Autodesk Inventor part; units mm, degrees
(part 9 of 16)
  spline S53 degree 3 poles (39.1598, 73.1537) (39.0289, 73.1211) (38.8976, 73.0905) (38.7657, 73.0621) (38.6945, 73.0467) (38.6231, 73.0319) (38.5516, 73.0177) (38.4838, 73.0044) (38.416, 72.9916) (38.3481, 72.9794) (38.284, 72.9679) (38.2197, 72.957) (38.1554, 72.9466) (38.095, 72.9369) (38.0344, 72.9277) (37.9738, 72.919) (37.917, 72.9109) (37.8601, 72.9033) (37.8032, 72.8962) (37.7501, 72.8896) (37.697, 72.8834) (37.6438, 72.8778) (37.5945, 72.8725) (37.5452, 72.8677) (37.4958, 72.8633) (37.4502, 72.8593) (37.4047, 72.8556) (37.3591, 72.8524) (37.3174, 72.8494) (37.2756, 72.8469) (37.2339, 72.8446) (37.196, 72.8426) (37.1581, 72.841) (37.1202, 72.8396) (37.0861, 72.8384) (37.0521, 72.8375) (37.0181, 72.8369) (36.9731, 72.8362) (36.9281, 72.8361) (36.8831, 72.8364) (36.873, 72.8364) (36.863, 72.8365) (36.8529, 72.8365) (36.8431, 72.8364) (36.8332, 72.8363) (36.8234, 72.8361) (36.8138, 72.8359) (36.8041, 72.8356) (36.7945, 72.8352) (36.7851, 72.8348) (36.7757, 72.8344) (36.7662, 72.8338) (36.757, 72.8333) (36.7477, 72.8327) (36.7385, 72.8319) (36.7294, 72.8312) (36.7203, 72.8304) (36.7113, 72.8295) (36.7023, 72.8286) (36.6933, 72.8276) (36.6844, 72.8265) (36.6756, 72.8254) (36.6667, 72.8242) (36.6579, 72.8229) (36.6491, 72.8216) (36.6403, 72.8201) (36.6316, 72.8186) (36.6228, 72.817) (36.6141, 72.8153) (36.6054, 72.8135) (36.5966, 72.8116) (36.5878, 72.8097) (36.5791, 72.8075) (36.5702, 72.8053) (36.5613, 72.803) (36.5525, 72.8005) (36.5435, 72.7979) (36.5345, 72.7952) (36.5255, 72.7922) (36.5162, 72.7892) (36.507, 72.7859) (36.4978, 72.7824) (36.4882, 72.7787) (36.4786, 72.7748) (36.4692, 72.7706) (36.459, 72.7661) (36.449, 72.7613) (36.4392, 72.7562) (36.4285, 72.7507) (36.418, 72.7448) (36.4078, 72.7385) (36.3964, 72.7316) (36.3854, 72.7242) (36.3747, 72.7164) (36.3627, 72.7077) (36.3511, 72.6984) (36.3401, 72.6885) (36.3276, 72.6775) (36.3157, 72.6658) (36.3046, 72.6534) (36.2921, 72.6395) (36.2804, 72.6248) (36.2698, 72.6094) (36.258, 72.5923) (36.2474, 72.5743) (36.2382, 72.5556) (36.2281, 72.5354) (36.2197, 72.5143) (36.2132, 72.4928) (36.207, 72.4721) (36.2027, 72.451) (36.1987, 72.4298) (36.1788, 72.3251) (36.168, 72.219) (36.1519, 72.1138) (36.1359, 72.0085) (36.1147, 71.904) (36.1024, 71.7981) (36.0999, 71.7767) (36.0978, 71.7552) (36.0976, 71.7337) (36.0973, 71.7112) (36.0991, 71.6886) (36.1026, 71.6663) (36.1059, 71.6457) (36.1106, 71.6254) (36.1168, 71.6055) (36.1224, 71.5877) (36.1291, 71.5702) (36.1369, 71.5532) (36.1439, 71.538) (36.1517, 71.5233) (36.1603, 71.509) (36.168, 71.4963) (36.1763, 71.484) (36.1851, 71.4721) (36.193, 71.4615) (36.2013, 71.4511) (36.2101, 71.4412) (36.218, 71.4321) (36.2263, 71.4234) (36.2348, 71.4149) (36.2427, 71.4071) (36.2508, 71.3995) (36.2591, 71.3922) (36.2669, 71.3854) (36.2749, 71.3788) (36.283, 71.3724) (36.2907, 71.3664) (36.2985, 71.3605) (36.3065, 71.3548) (36.3142, 71.3493) (36.3219, 71.344) (36.3298, 71.3389) (36.3375, 71.3338) (36.3452, 71.329) (36.3531, 71.3243) (36.3608, 71.3196) (36.3685, 71.3151) (36.3764, 71.3107) (36.3842, 71.3064) (36.392, 71.3022) (36.3999, 71.2981) (36.4078, 71.294) (36.4157, 71.29) (36.4237, 71.2861) (36.4318, 71.2822) (36.4398, 71.2785) (36.448, 71.2748) (36.4562, 71.2711) (36.4644, 71.2674) (36.4727, 71.2639) (36.4811, 71.2603) (36.4895, 71.2569) (36.498, 71.2535) (36.5066, 71.25) (36.5152, 71.2467) (36.5239, 71.2434) (36.5327, 71.2401) (36.5416, 71.2368) (36.5505, 71.2337) (36.5595, 71.2304) (36.5686, 71.2273) (36.5778, 71.2242) (36.5871, 71.2211) (36.5965, 71.218) (36.6058, 71.2151) (36.6154, 71.2121) (36.6251, 71.2091) (36.6347, 71.2062) (36.6777, 71.193) (36.7207, 71.1795) (36.7634, 71.1654) (36.7957, 71.1548) (36.8279, 71.1437) (36.86, 71.1325) (36.8958, 71.1199) (36.9315, 71.107) (36.9671, 71.0938) (37.0063, 71.0793) (37.0454, 71.0643) (37.0843, 71.0491) (37.1269, 71.0324) (37.1693, 71.0154) (37.2115, 70.998) (37.2574, 70.9791) (37.3031, 70.9598) (37.3486, 70.9401) (37.3976, 70.9188) (37.4465, 70.8971) (37.4952, 70.875) (37.5474, 70.8513) (37.5995, 70.8271) (37.6512, 70.8024) (37.7066, 70.7761) (37.7616, 70.7493) (37.8165, 70.722) (37.8748, 70.693) (37.9328, 70.6634) (37.9906, 70.6333) (38.0518, 70.6015) (38.1128, 70.5691) (38.1734, 70.5361) (38.2375, 70.5013) (38.3012, 70.4659) (38.3647, 70.43) (38.482, 70.3636) (38.5983, 70.2952) (38.7136, 70.2252) knots 0 0 0 0 0.057795 0.057795 0.057795 0.089038 0.089038 0.089038 0.118617 0.118617 0.118617 0.14653 0.14653 0.14653 0.172778 0.172778 0.172778 0.19736 0.19736 0.19736 0.220277 0.220277 0.220277 0.241529 0.241529 0.241529 0.261115 0.261115 0.261115 0.279036 0.279036 0.279036 0.295292 0.295292 0.295292 0.309882 0.309882 0.309882 0.329164 0.329164 0.329164 0.333477 0.333477 0.333477 0.337694 0.337694 0.337694 0.34182 0.34182 0.34182 0.345864 0.345864 0.345864 0.349834 0.349834 0.349834 0.353742 0.353742 0.353742 0.3576 0.3576 0.3576 0.361424 0.361424 0.361424 0.365232 0.365232 0.365232 0.369048 0.369048 0.369048 0.372899 0.372899 0.372899 0.376819 0.376819 0.376819 0.380853 0.380853 0.380853 0.385052 0.385052 0.385052 0.389482 0.389482 0.389482 0.394225 0.394225 0.394225 0.399381 0.399381 0.399381 0.405067 0.405067 0.405067 0.411413 0.411413 0.411413 0.418548 0.418548 0.418548 0.426565 0.426565 0.426565 0.435472 0.435472 0.435472 0.445133 0.445133 0.445133 0.45436 0.45436 0.45436 0.5 0.5 0.5 0.54564 0.54564 0.54564 0.554867 0.554867 0.554867 0.564528 0.564528 0.564528 0.573435 0.573435 0.573435 0.581452 0.581452 0.581452 0.588587 0.588587 0.588587 0.594933 0.594933 0.594933 0.600619 0.600619 0.600619 0.605775 0.605775 0.605775 0.610518 0.610518 0.610518 0.614948 0.614948 0.614948 0.619147 0.619147 0.619147 0.623181 0.623181 0.623181 0.627101 0.627101 0.627101 0.630952 0.630952 0.630952 0.634768 0.634768 0.634768 0.638576 0.638576 0.638576 0.6424 0.6424 0.6424 0.646258 0.646258 0.646258 0.650166 0.650166 0.650166 0.654136 0.654136 0.654136 0.65818 0.65818 0.65818 0.662306 0.662306 0.662306 0.666523 0.666523 0.666523 0.670836 0.670836 0.670836 0.690118 0.690118 0.690118 0.704708 0.704708 0.704708 0.720964 0.720964 0.720964 0.738885 0.738885 0.738885 0.758471 0.758471 0.758471 0.779723 0.779723 0.779723 0.80264 0.80264 0.80264 0.827222 0.827222 0.827222 0.85347 0.85347 0.85347 0.881383 0.881383 0.881383 0.910962 0.910962 0.910962 0.942205 0.942205 0.942205 1 1 1 1
  arc A255 (39.1598, 73.1537) -> (39.2743, 74.3078) centre (0.0435, 77.6158) ccw
  spline S54 degree 3 poles (39.4119, 77.2669) (39.2852, 77.2209) (39.1577, 77.1767) (39.0296, 77.1346) (38.9603, 77.1118) (38.8909, 77.0896) (38.8212, 77.0681) (38.7553, 77.0477) (38.6892, 77.0279) (38.6229, 77.0087) (38.5603, 76.9906) (38.4976, 76.973) (38.4347, 76.956) (38.3756, 76.94) (38.3163, 76.9245) (38.2569, 76.9096) (38.2013, 76.8956) (38.1455, 76.882) (38.0897, 76.869) (38.0376, 76.8569) (37.9854, 76.8452) (37.9331, 76.834) (37.8846, 76.8237) (37.836, 76.8137) (37.7874, 76.8042) (37.7425, 76.7954) (37.6976, 76.787) (37.6526, 76.779) (37.6114, 76.7717) (37.5701, 76.7648) (37.5288, 76.7582) (37.4914, 76.7523) (37.4539, 76.7467) (37.4163, 76.7414) (37.3826, 76.7366) (37.3488, 76.7321) (37.315, 76.728) (37.2704, 76.7226) (37.2256, 76.7178) (37.1809, 76.7133) (37.1708, 76.7123) (37.1608, 76.7114) (37.1508, 76.7103) (37.141, 76.7092) (37.1313, 76.708) (37.1215, 76.7068) (37.112, 76.7056) (37.1024, 76.7043) (37.0929, 76.7029) (37.0835, 76.7016) (37.0742, 76.7001) (37.0649, 76.6986) (37.0558, 76.6971) (37.0466, 76.6955) (37.0375, 76.6938) (37.0286, 76.6922) (37.0196, 76.6904) (37.0107, 76.6885) (37.0019, 76.6867) (36.9931, 76.6848) (36.9843, 76.6828) (36.9756, 76.6807) (36.9669, 76.6786) (36.9583, 76.6764) (36.9497, 76.6741) (36.9411, 76.6718) (36.9326, 76.6693) (36.924, 76.6669) (36.9155, 76.6643) (36.907, 76.6615) (36.8985, 76.6588) (36.89, 76.6559) (36.8815, 76.6529) (36.8729, 76.6498) (36.8644, 76.6465) (36.8559, 76.6431) (36.8471, 76.6396) (36.8385, 76.6359) (36.8299, 76.6321) (36.8209, 76.6281) (36.8121, 76.6238) (36.8034, 76.6194) (36.7941, 76.6147) (36.785, 76.6098) (36.7761, 76.6047) (36.7665, 76.5991) (36.757, 76.5933) (36.7478, 76.5872) (36.7378, 76.5806) (36.7279, 76.5736) (36.7184, 76.5663) (36.7078, 76.5583) (36.6976, 76.5498) (36.6878, 76.5409) (36.6768, 76.5309) (36.6663, 76.5205) (36.6563, 76.5096) (36.645, 76.4973) (36.6345, 76.4844) (36.6247, 76.4709) (36.6136, 76.4557) (36.6036, 76.4399) (36.5946, 76.4235) (36.5847, 76.4052) (36.576, 76.3862) (36.5688, 76.3667) (36.561, 76.3455) (36.5548, 76.3237) (36.5506, 76.3016) (36.5466, 76.2804) (36.5444, 76.259) (36.5427, 76.2375) (36.5339, 76.1312) (36.5342, 76.0246) (36.5292, 75.9183) (36.5243, 75.8119) (36.5141, 75.7058) (36.513, 75.5992) (36.5127, 75.5776) (36.5129, 75.556) (36.5149, 75.5346) (36.517, 75.5122) (36.5212, 75.4899) (36.527, 75.4681) (36.5324, 75.448) (36.5392, 75.4283) (36.5474, 75.4092) (36.5548, 75.392) (36.5634, 75.3753) (36.5729, 75.3592) (36.5814, 75.3448) (36.5908, 75.331) (36.6008, 75.3177) (36.6097, 75.3059) (36.6193, 75.2945) (36.6293, 75.2836) (36.6383, 75.2738) (36.6476, 75.2644) (36.6574, 75.2554) (36.6662, 75.2473) (36.6754, 75.2394) (36.6847, 75.2319) (36.6934, 75.2249) (36.7022, 75.2183) (36.7113, 75.2119) (36.7197, 75.2059) (36.7283, 75.2002) (36.7371, 75.1947) (36.7454, 75.1895) (36.7538, 75.1844) (36.7623, 75.1796) (36.7705, 75.175) (36.7788, 75.1705) (36.7871, 75.1662) (36.7953, 75.162) (36.8035, 75.158) (36.8118, 75.1541) (36.8199, 75.1503) (36.8281, 75.1466) (36.8364, 75.1431) (36.8446, 75.1396) (36.8528, 75.1362) (36.8611, 75.133) (36.8694, 75.1297) (36.8777, 75.1266) (36.8861, 75.1236) (36.8945, 75.1205) (36.9029, 75.1176) (36.9114, 75.1148) (36.9199, 75.112) (36.9285, 75.1092) (36.9371, 75.1066) (36.9458, 75.1039) (36.9545, 75.1013) (36.9633, 75.0989) (36.9722, 75.0963) (36.9812, 75.0939) (36.9901, 75.0916) (36.9993, 75.0892) (37.0084, 75.0869) (37.0176, 75.0847) (37.027, 75.0824) (37.0363, 75.0802) (37.0457, 75.0781) (37.0553, 75.076) (37.065, 75.0739) (37.0746, 75.072) (37.0845, 75.0699) (37.0943, 75.068) (37.1042, 75.0661) (37.1484, 75.0575) (37.1925, 75.0486) (37.2365, 75.039) (37.2697, 75.0318) (37.3029, 75.0242) (37.3361, 75.0163) (37.373, 75.0076) (37.4098, 74.9985) (37.4465, 74.9891) (37.4871, 74.9787) (37.5275, 74.968) (37.5678, 74.9569) (37.6119, 74.9448) (37.6558, 74.9323) (37.6997, 74.9194) (37.7472, 74.9054) (37.7947, 74.8909) (37.842, 74.8761) (37.893, 74.8601) (37.9439, 74.8436) (37.9946, 74.8267) (38.0491, 74.8086) (38.1033, 74.7899) (38.1574, 74.7708) (38.2152, 74.7504) (38.2727, 74.7295) (38.3301, 74.7081) (38.3911, 74.6853) (38.452, 74.662) (38.5126, 74.6381) (38.5768, 74.6128) (38.6408, 74.587) (38.7046, 74.5606) (38.7719, 74.5327) (38.839, 74.5041) (38.9059, 74.475) (39.0295, 74.4212) (39.1523, 74.3654) (39.2743, 74.3078) knots 0 0 0 0 0.057795 0.057795 0.057795 0.089038 0.089038 0.089038 0.118617 0.118617 0.118617 0.14653 0.14653 0.14653 0.172778 0.172778 0.172778 0.19736 0.19736 0.19736 0.220277 0.220277 0.220277 0.241529 0.241529 0.241529 0.261115 0.261115 0.261115 0.279036 0.279036 0.279036 0.295292 0.295292 0.295292 0.309882 0.309882 0.309882 0.329164 0.329164 0.329164 0.333477 0.333477 0.333477 0.337694 0.337694 0.337694 0.34182 0.34182 0.34182 0.345864 0.345864 0.345864 0.349834 0.349834 0.349834 0.353742 0.353742 0.353742 0.3576 0.3576 0.3576 0.361424 0.361424 0.361424 0.365232 0.365232 0.365232 0.369048 0.369048 0.369048 0.372899 0.372899 0.372899 0.376819 0.376819 0.376819 0.380853 0.380853 0.380853 0.385052 0.385052 0.385052 0.389482 0.389482 0.389482 0.394225 0.394225 0.394225 0.399381 0.399381 0.399381 0.405067 0.405067 0.405067 0.411413 0.411413 0.411413 0.418548 0.418548 0.418548 0.426565 0.426565 0.426565 0.435472 0.435472 0.435472 0.445133 0.445133 0.445133 0.45436 0.45436 0.45436 0.5 0.5 0.5 0.54564 0.54564 0.54564 0.554867 0.554867 0.554867 0.564528 0.564528 0.564528 0.573435 0.573435 0.573435 0.581452 0.581452 0.581452 0.588587 0.588587 0.588587 0.594933 0.594933 0.594933 0.600619 0.600619 0.600619 0.605775 0.605775 0.605775 0.610518 0.610518 0.610518 0.614948 0.614948 0.614948 0.619147 0.619147 0.619147 0.623181 0.623181 0.623181 0.627101 0.627101 0.627101 0.630952 0.630952 0.630952 0.634768 0.634768 0.634768 0.638576 0.638576 0.638576 0.6424 0.6424 0.6424 0.646258 0.646258 0.646258 0.650166 0.650166 0.650166 0.654136 0.654136 0.654136 0.65818 0.65818 0.65818 0.662306 0.662306 0.662306 0.666523 0.666523 0.666523 0.670836 0.670836 0.670836 0.690118 0.690118 0.690118 0.704708 0.704708 0.704708 0.720964 0.720964 0.720964 0.738885 0.738885 0.738885 0.758471 0.758471 0.758471 0.779723 0.779723 0.779723 0.80264 0.80264 0.80264 0.827222 0.827222 0.827222 0.85347 0.85347 0.85347 0.881383 0.881383 0.881383 0.910962 0.910962 0.910962 0.942205 0.942205 0.942205 1 1 1 1
  arc A256 (39.4119, 77.2669) -> (39.4051, 78.4267) centre (0.0435, 77.6158) ccw
  spline S55 degree 3 poles (39.2328, 81.3839) (39.1115, 81.3249) (38.9894, 81.2676) (38.8663, 81.2124) (38.7998, 81.1825) (38.7331, 81.1532) (38.666, 81.1245) (38.6026, 81.0973) (38.5389, 81.0707) (38.475, 81.0447) (38.4147, 81.0201) (38.3541, 80.9961) (38.2934, 80.9726) (38.2362, 80.9505) (38.1789, 80.9289) (38.1214, 80.9078) (38.0675, 80.8881) (38.0135, 80.8688) (37.9593, 80.85) (37.9088, 80.8325) (37.8581, 80.8155) (37.8073, 80.7989) (37.7601, 80.7835) (37.7128, 80.7685) (37.6654, 80.7539) (37.6217, 80.7405) (37.5779, 80.7275) (37.534, 80.7148) (37.4938, 80.7033) (37.4535, 80.6921) (37.4131, 80.6812) (37.3765, 80.6714) (37.3398, 80.6619) (37.303, 80.6527) (37.2699, 80.6444) (37.2368, 80.6364) (37.2037, 80.6288) (37.1598, 80.6187) (37.1158, 80.6093) (37.0718, 80.6002) (37.0619, 80.5981) (37.052, 80.5961) (37.0422, 80.594) (37.0326, 80.5919) (37.023, 80.5897) (37.0134, 80.5875) (37.004, 80.5853) (36.9947, 80.583) (36.9853, 80.5806) (36.9762, 80.5783) (36.9671, 80.5759) (36.958, 80.5734) (36.949, 80.571) (36.9401, 80.5684) (36.9312, 80.5658) (36.9225, 80.5632) (36.9138, 80.5605) (36.9051, 80.5578) (36.8965, 80.555) (36.888, 80.5522) (36.8795, 80.5492) (36.871, 80.5463) (36.8626, 80.5433) (36.8543, 80.5402) (36.846, 80.5371) (36.8377, 80.5338) (36.8294, 80.5305) (36.8212, 80.5271) (36.813, 80.5237) (36.8048, 80.5201) (36.7966, 80.5164) (36.7885, 80.5127) (36.7804, 80.5088) (36.7721, 80.5048) (36.764, 80.5007) (36.7559, 80.4964) (36.7475, 80.492) (36.7393, 80.4874) (36.7312, 80.4827) (36.7227, 80.4778) (36.7144, 80.4726) (36.7061, 80.4673) (36.6974, 80.4617) (36.6889, 80.4559) (36.6805, 80.4498) (36.6716, 80.4433) (36.6628, 80.4365) (36.6542, 80.4295) (36.6449, 80.4219) (36.6359, 80.4139) (36.6272, 80.4056) (36.6175, 80.3965) (36.6083, 80.387) (36.5994, 80.3771) (36.5895, 80.3661) (36.5801, 80.3546) (36.5713, 80.3427) (36.5614, 80.3293) (36.5523, 80.3154) (36.5439, 80.3009) (36.5346, 80.2847) (36.5262, 80.2679) (36.519, 80.2506) (36.511, 80.2314) (36.5044, 80.2117) (36.4993, 80.1915) (36.4937, 80.1696) (36.4898, 80.1473) (36.488, 80.1248) (36.4862, 80.1034) (36.4863, 80.0818) (36.4868, 80.0602) (36.4892, 79.9536) (36.5006, 79.8476) (36.5068, 79.7414) (36.513, 79.6351) (36.514, 79.5285) (36.524, 79.4223) (36.526, 79.4009) (36.5284, 79.3794) (36.5326, 79.3583) (36.5371, 79.3362) (36.5435, 79.3145) (36.5516, 79.2934) (36.5591, 79.274) (36.5679, 79.2551) (36.5781, 79.2369) (36.5873, 79.2206) (36.5975, 79.2049) (36.6087, 79.1899) (36.6187, 79.1765) (36.6294, 79.1637) (36.6408, 79.1516) (36.6509, 79.1408) (36.6615, 79.1304) (36.6726, 79.1206) (36.6826, 79.1119) (36.6929, 79.1035) (36.7035, 79.0955) (36.7132, 79.0883) (36.7231, 79.0815) (36.7332, 79.075) (36.7425, 79.069) (36.752, 79.0633) (36.7617, 79.0579) (36.7707, 79.0528) (36.7799, 79.048) (36.7891, 79.0435) (36.7979, 79.0391) (36.8068, 79.035) (36.8158, 79.0311) (36.8244, 79.0273) (36.8331, 79.0238) (36.8419, 79.0204) (36.8504, 79.0171) (36.859, 79.0139) (36.8677, 79.0109) (36.8762, 79.008) (36.8847, 79.0052) (36.8933, 79.0026) (36.9018, 78.9999) (36.9104, 78.9974) (36.9189, 78.9951) (36.9275, 78.9927) (36.9361, 78.9905) (36.9447, 78.9883) (36.9534, 78.9862) (36.9621, 78.9842) (36.9708, 78.9823) (36.9796, 78.9803) (36.9884, 78.9785) (36.9973, 78.9768) (37.0062, 78.975) (37.0152, 78.9734) (37.0242, 78.9718) (37.0333, 78.9702) (37.0424, 78.9688) (37.0516, 78.9674) (37.0609, 78.9659) (37.0703, 78.9646) (37.0796, 78.9634) (37.0892, 78.9621) (37.0987, 78.9609) (37.1083, 78.9598) (37.1181, 78.9587) (37.1278, 78.9576) (37.1376, 78.9567) (37.1477, 78.9557) (37.1577, 78.9549) (37.1677, 78.954) (37.2125, 78.9501) (37.2573, 78.9458) (37.3021, 78.9409) (37.3359, 78.9372) (37.3697, 78.9331) (37.4035, 78.9287) (37.4411, 78.9239) (37.4787, 78.9187) (37.5162, 78.9132) (37.5576, 78.9071) (37.5989, 78.9006) (37.6402, 78.8938) (37.6853, 78.8864) (37.7303, 78.8785) (37.7752, 78.8703) (37.824, 78.8613) (37.8727, 78.8519) (37.9213, 78.8421) (37.9737, 78.8315) (38.0261, 78.8205) (38.0783, 78.809) (38.1343, 78.7966) (38.1902, 78.7837) (38.246, 78.7704) (38.3056, 78.7562) (38.365, 78.7414) (38.4243, 78.7261) (38.4874, 78.7098) (38.5503, 78.6929) (38.6131, 78.6756) (38.6796, 78.6571) (38.746, 78.6381) (38.8121, 78.6185) (38.882, 78.5978) (38.9517, 78.5764) (39.0213, 78.5545) (39.1499, 78.5139) (39.2778, 78.4712) (39.4051, 78.4267) knots 0 0 0 0 0.057795 0.057795 0.057795 0.089038 0.089038 0.089038 0.118617 0.118617 0.118617 0.14653 0.14653 0.14653 0.172778 0.172778 0.172778 0.19736 0.19736 0.19736 0.220277 0.220277 0.220277 0.241529 0.241529 0.241529 0.261115 0.261115 0.261115 0.279036 0.279036 0.279036 0.295292 0.295292 0.295292 0.309882 0.309882 0.309882 0.329164 0.329164 0.329164 0.333477 0.333477 0.333477 0.337694 0.337694 0.337694 0.34182 0.34182 0.34182 0.345864 0.345864 0.345864 0.349834 0.349834 0.349834 0.353742 0.353742 0.353742 0.3576 0.3576 0.3576 0.361424 0.361424 0.361424 0.365232 0.365232 0.365232 0.369048 0.369048 0.369048 0.372899 0.372899 0.372899 0.376819 0.376819 0.376819 0.380853 0.380853 0.380853 0.385052 0.385052 0.385052 0.389482 0.389482 0.389482 0.394225 0.394225 0.394225 0.399381 0.399381 0.399381 0.405067 0.405067 0.405067 0.411413 0.411413 0.411413 0.418548 0.418548 0.418548 0.426565 0.426565 0.426565 0.435472 0.435472 0.435472 0.445133 0.445133 0.445133 0.45436 0.45436 0.45436 0.5 0.5 0.5 0.54564 0.54564 0.54564 0.554867 0.554867 0.554867 0.564528 0.564528 0.564528 0.573435 0.573435 0.573435 0.581452 0.581452 0.581452 0.588587 0.588587 0.588587 0.594933 0.594933 0.594933 0.600619 0.600619 0.600619 0.605775 0.605775 0.605775 0.610518 0.610518 0.610518 0.614948 0.614948 0.614948 0.619147 0.619147 0.619147 0.623181 0.623181 0.623181 0.627101 0.627101 0.627101 0.630952 0.630952 0.630952 0.634768 0.634768 0.634768 0.638576 0.638576 0.638576 0.6424 0.6424 0.6424 0.646258 0.646258 0.646258 0.650166 0.650166 0.650166 0.654136 0.654136 0.654136 0.65818 0.65818 0.65818 0.662306 0.662306 0.662306 0.666523 0.666523 0.666523 0.670836 0.670836 0.670836 0.690118 0.690118 0.690118 0.704708 0.704708 0.704708 0.720964 0.720964 0.720964 0.738885 0.738885 0.738885 0.758471 0.758471 0.758471 0.779723 0.779723 0.779723 0.80264 0.80264 0.80264 0.827222 0.827222 0.827222 0.85347 0.85347 0.85347 0.881383 0.881383 0.881383 0.910962 0.910962 0.910962 0.942205 0.942205 0.942205 1 1 1 1
  arc A257 (39.2328, 81.3839) -> (39.1048, 82.5366) centre (0.0435, 77.6158) ccw
  spline S56 degree 3 poles (38.6242, 85.4597) (38.5098, 85.3883) (38.3943, 85.3186) (38.2777, 85.2508) (38.2147, 85.2141) (38.1514, 85.178) (38.0877, 85.1424) (38.0274, 85.1088) (37.9669, 85.0756) (37.906, 85.0431) (37.8486, 85.0123) (37.7909, 84.9821) (37.7329, 84.9524) (37.6784, 84.9244) (37.6237, 84.897) (37.5687, 84.87) (37.5172, 84.8447) (37.4655, 84.8199) (37.4135, 84.7956) (37.3651, 84.7729) (37.3165, 84.7506) (37.2677, 84.7288) (37.2224, 84.7086) (37.1769, 84.6887) (37.1313, 84.6693) (37.0893, 84.6514) (37.047, 84.6338) (37.0047, 84.6167) (36.9659, 84.601) (36.927, 84.5856) (36.888, 84.5706) (36.8526, 84.557) (36.8171, 84.5437) (36.7814, 84.5307) (36.7494, 84.5191) (36.7173, 84.5077) (36.6851, 84.4966) (36.6426, 84.482) (36.5998, 84.468) (36.557, 84.4543) (36.5474, 84.4513) (36.5378, 84.4482) (36.5282, 84.4451) (36.5189, 84.442) (36.5095, 84.4389) (36.5003, 84.4356) (36.4912, 84.4324) (36.4821, 84.4292) (36.4731, 84.4259) (36.4642, 84.4226) (36.4554, 84.4193) (36.4466, 84.4158) (36.438, 84.4125) (36.4294, 84.409) (36.4208, 84.4055) (36.4124, 84.402) (36.404, 84.3984) (36.3956, 84.3947) (36.3874, 84.3911) (36.3792, 84.3874) (36.371, 84.3836) (36.363, 84.3798) (36.3549, 84.3759) (36.3469, 84.3719) (36.339, 84.368) (36.3311, 84.3639) (36.3233, 84.3597) (36.3154, 84.3555) (36.3076, 84.3512) (36.2999, 84.3468) (36.2921, 84.3423) (36.2844, 84.3377) (36.2767, 84.333) (36.2689, 84.3282) (36.2612, 84.3232) (36.2536, 84.3181) (36.2458, 84.3129) (36.2381, 84.3075) (36.2305, 84.3019) (36.2226, 84.2961) (36.2148, 84.2901) (36.2072, 84.284) (36.1992, 84.2775) (36.1913, 84.2708) (36.1836, 84.2639) (36.1754, 84.2565) (36.1673, 84.2489) (36.1596, 84.241) (36.1511, 84.2324) (36.143, 84.2235) (36.1351, 84.2144) (36.1265, 84.2043) (36.1183, 84.1939) (36.1105, 84.1831) (36.1018, 84.1711) (36.0937, 84.1587) (36.0862, 84.146) (36.0777, 84.1316) (36.0701, 84.1168) (36.0633, 84.1016) (36.0557, 84.0845) (36.0491, 84.0669) (36.0438, 84.0489) (36.0378, 84.029) (36.0334, 84.0086) (36.0303, 83.988) (36.0271, 83.9657) (36.0255, 83.9431) (36.026, 83.9206) (36.0265, 83.899) (36.0289, 83.8776) (36.0316, 83.8562) (36.0452, 83.7504) (36.0676, 83.6462) (36.0849, 83.5412) (36.1021, 83.4361) (36.1143, 83.3302) (36.1353, 83.2257) (36.1396, 83.2045) (36.1442, 83.1835) (36.1506, 83.1629) (36.1573, 83.1414) (36.166, 83.1205) (36.1763, 83.1003) (36.1857, 83.0818) (36.1965, 83.0639) (36.2085, 83.047) (36.2193, 83.0317) (36.2312, 83.0171) (36.2439, 83.0034) (36.2552, 82.9911) (36.2672, 82.9795) (36.2797, 82.9686) (36.2909, 82.9589) (36.3026, 82.9498) (36.3147, 82.9412) (36.3255, 82.9335) (36.3366, 82.9262) (36.348, 82.9195) (36.3584, 82.9133) (36.3689, 82.9075) (36.3797, 82.9021) (36.3896, 82.8971) (36.3996, 82.8925) (36.4098, 82.8881) (36.4193, 82.884) (36.4289, 82.8802) (36.4386, 82.8766) (36.4478, 82.8732) (36.4571, 82.8701) (36.4664, 82.8671) (36.4754, 82.8643) (36.4844, 82.8616) (36.4935, 82.8592) (36.5023, 82.8568) (36.5112, 82.8545) (36.5201, 82.8525) (36.5289, 82.8504) (36.5377, 82.8486) (36.5465, 82.8468) (36.5552, 82.8451) (36.564, 82.8435) (36.5728, 82.842) (36.5815, 82.8406) (36.5903, 82.8393) (36.5991, 82.838) (36.608, 82.8368) (36.6168, 82.8357) (36.6257, 82.8347) (36.6346, 82.8337) (36.6436, 82.8328) (36.6526, 82.832) (36.6616, 82.8312) (36.6707, 82.8305) (36.6798, 82.8299) (36.6891, 82.8293) (36.6983, 82.8288) (36.7076, 82.8284) (36.717, 82.8279) (36.7264, 82.8276) (36.7359, 82.8273) (36.7455, 82.827) (36.7551, 82.8269) (36.7648, 82.8268) (36.7746, 82.8267) (36.7844, 82.8267) (36.7943, 82.8267) (36.8043, 82.8268) (36.8144, 82.827) (36.8245, 82.8272) (36.8695, 82.828) (36.9144, 82.8284) (36.9594, 82.8282) (36.9935, 82.828) (37.0275, 82.8275) (37.0616, 82.8267) (37.0995, 82.8258) (37.1374, 82.8246) (37.1753, 82.823) (37.2171, 82.8213) (37.2589, 82.8192) (37.3006, 82.8167) (37.3462, 82.814) (37.3918, 82.8109) (37.4374, 82.8074) (37.4869, 82.8036) (37.5363, 82.7994) (37.5856, 82.7947) (37.6389, 82.7897) (37.6921, 82.7841) (37.7452, 82.7781) (37.8022, 82.7717) (37.8592, 82.7648) (37.916, 82.7573) (37.9768, 82.7494) (38.0374, 82.7409) (38.098, 82.7319) (38.1624, 82.7223) (38.2268, 82.7121) (38.291, 82.7014) (38.3591, 82.69) (38.4271, 82.678) (38.4949, 82.6654) (38.5666, 82.6521) (38.6382, 82.6382) (38.7096, 82.6236) (38.8418, 82.5967) (38.9735, 82.5676) (39.1048, 82.5366) knots 0 0 0 0 0.057795 0.057795 0.057795 0.089038 0.089038 0.089038 0.118617 0.118617 0.118617 0.14653 0.14653 0.14653 0.172778 0.172778 0.172778 0.19736 0.19736 0.19736 0.220277 0.220277 0.220277 0.241529 0.241529 0.241529 0.261115 0.261115 0.261115 0.279036 0.279036 0.279036 0.295292 0.295292 0.295292 0.309882 0.309882 0.309882 0.329164 0.329164 0.329164 0.333477 0.333477 0.333477 0.337694 0.337694 0.337694 0.34182 0.34182 0.34182 0.345864 0.345864 0.345864 0.349834 0.349834 0.349834 0.353742 0.353742 0.353742 0.3576 0.3576 0.3576 0.361424 0.361424 0.361424 0.365232 0.365232 0.365232 0.369048 0.369048 0.369048 0.372899 0.372899 0.372899 0.376819 0.376819 0.376819 0.380853 0.380853 0.380853 0.385052 0.385052 0.385052 0.389482 0.389482 0.389482 0.394225 0.394225 0.394225 0.399381 0.399381 0.399381 0.405067 0.405067 0.405067 0.411413 0.411413 0.411413 0.418548 0.418548 0.418548 0.426565 0.426565 0.426565 0.435472 0.435472 0.435472 0.445133 0.445133 0.445133 0.45436 0.45436 0.45436 0.5 0.5 0.5 0.54564 0.54564 0.54564 0.554867 0.554867 0.554867 0.564528 0.564528 0.564528 0.573435 0.573435 0.573435 0.581452 0.581452 0.581452 0.588587 0.588587 0.588587 0.594933 0.594933 0.594933 0.600619 0.600619 0.600619 0.605775 0.605775 0.605775 0.610518 0.610518 0.610518 0.614948 0.614948 0.614948 0.619147 0.619147 0.619147 0.623181 0.623181 0.623181 0.627101 0.627101 0.627101 0.630952 0.630952 0.630952 0.634768 0.634768 0.634768 0.638576 0.638576 0.638576 0.6424 0.6424 0.6424 0.646258 0.646258 0.646258 0.650166 0.650166 0.650166 0.654136 0.654136 0.654136 0.65818 0.65818 0.65818 0.662306 0.662306 0.662306 0.666523 0.666523 0.666523 0.670836 0.670836 0.670836 0.690118 0.690118 0.690118 0.704708 0.704708 0.704708 0.720964 0.720964 0.720964 0.738885 0.738885 0.738885 0.758471 0.758471 0.758471 0.779723 0.779723 0.779723 0.80264 0.80264 0.80264 0.827222 0.827222 0.827222 0.85347 0.85347 0.85347 0.881383 0.881383 0.881383 0.910962 0.910962 0.910962 0.942205 0.942205 0.942205 1 1 1 1
  arc A258 (38.6242, 85.4597) -> (38.3764, 86.5927) centre (0.0435, 77.6158) ccw
  spline S57 degree 3 poles (37.5929, 89.4495) (37.4866, 89.3665) (37.379, 89.2851) (37.2702, 89.2055) (37.2114, 89.1624) (37.1521, 89.1199) (37.0925, 89.0779) (37.0361, 89.0381) (36.9794, 88.9989) (36.9223, 88.9601) (36.8684, 88.9235) (36.8141, 88.8874) (36.7596, 88.8518) (36.7083, 88.8183) (36.6567, 88.7853) (36.6049, 88.7527) (36.5563, 88.7222) (36.5074, 88.6921) (36.4583, 88.6625) (36.4125, 88.6349) (36.3665, 88.6076) (36.3202, 88.5808) (36.2773, 88.556) (36.2342, 88.5315) (36.1908, 88.5074) (36.1509, 88.4852) (36.1108, 88.4633) (36.0704, 88.4418) (36.0335, 88.4222) (35.9964, 88.4028) (35.9592, 88.3838) (35.9254, 88.3666) (35.8914, 88.3496) (35.8574, 88.333) (35.8268, 88.3181) (35.796, 88.3034) (35.7652, 88.289) (35.7244, 88.27) (35.6833, 88.2516) (35.6421, 88.2336) (35.6329, 88.2295) (35.6237, 88.2255) (35.6145, 88.2214) (35.6055, 88.2174) (35.5966, 88.2132) (35.5877, 88.209) (35.579, 88.2049) (35.5703, 88.2007) (35.5616, 88.1965) (35.5532, 88.1923) (35.5448, 88.1881) (35.5364, 88.1837) (35.5281, 88.1795) (35.52, 88.1751) (35.5118, 88.1707) (35.5038, 88.1664) (35.4958, 88.1619) (35.4879, 88.1574) (35.4801, 88.153) (35.4723, 88.1484) (35.4646, 88.1438) (35.457, 88.1392) (35.4494, 88.1345) (35.4419, 88.1297) (35.4344, 88.1249) (35.4269, 88.12) (35.4196, 88.115) (35.4122, 88.11) (35.4049, 88.1049) (35.3977, 88.0997) (35.3904, 88.0945) (35.3832, 88.0891) (35.3761, 88.0836) (35.3689, 88.078) (35.3617, 88.0722) (35.3547, 88.0664) (35.3475, 88.0603) (35.3404, 88.0542) (35.3334, 88.0478) (35.3261, 88.0413) (35.319, 88.0345) (35.3121, 88.0276) (35.3048, 88.0203) (35.2976, 88.0128) (35.2907, 88.0051) (35.2833, 87.9969) (35.2761, 87.9885) (35.2692, 87.9798) (35.2617, 87.9704) (35.2545, 87.9608) (35.2477, 87.9509) (35.2401, 87.9399) (35.233, 87.9287) (35.2264, 87.9172) (35.2191, 87.9044) (35.2123, 87.8912) (35.2061, 87.8777) (35.1993, 87.8625) (35.1932, 87.847) (35.188, 87.8311) (35.1822, 87.8133) (35.1776, 87.7951) (35.1741, 87.7768) (35.1703, 87.7563) (35.168, 87.7356) (35.1671, 87.7148) (35.1662, 87.6922) (35.167, 87.6696) (35.1699, 87.6472) (35.1726, 87.6259) (35.1772, 87.6048) (35.1822, 87.5838) (35.2067, 87.48) (35.2399, 87.3787) (35.268, 87.2761) (35.2962, 87.1734) (35.3193, 87.0693) (35.3512, 86.9676) (35.3576, 86.947) (35.3644, 86.9265) (35.373, 86.9067) (35.3819, 86.8861) (35.3928, 86.8661) (35.4051, 86.8472) (35.4164, 86.8297) (35.429, 86.8131) (35.4427, 86.7975) (35.455, 86.7834) (35.4683, 86.7702) (35.4824, 86.7578) (35.4949, 86.7468) (35.508, 86.7366) (35.5217, 86.727) (35.5339, 86.7185) (35.5464, 86.7107) (35.5593, 86.7034) (35.5709, 86.6969) (35.5827, 86.6908) (35.5948, 86.6853) (35.6057, 86.6802) (35.6168, 86.6756) (35.6281, 86.6713) (35.6384, 86.6674) (35.6489, 86.6638) (35.6595, 86.6605) (35.6693, 86.6575) (35.6793, 86.6547) (35.6893, 86.6521) (35.6988, 86.6497) (35.7084, 86.6475) (35.718, 86.6456) (35.7272, 86.6437) (35.7365, 86.642) (35.7457, 86.6405) (35.7548, 86.639) (35.7638, 86.6377) (35.7729, 86.6366) (35.7818, 86.6355) (35.7908, 86.6346) (35.7997, 86.6338) (35.8086, 86.633) (35.8175, 86.6323) (35.8264, 86.6318) (35.8352, 86.6312) (35.8441, 86.6308) (35.853, 86.6305) (35.8619, 86.6302) (35.8708, 86.6301) (35.8798, 86.63) (35.8888, 86.63) (35.8978, 86.63) (35.9068, 86.6301) (35.9159, 86.6303) (35.925, 86.6305) (35.9341, 86.6309) (35.9434, 86.6312) (35.9526, 86.6317) (35.9619, 86.6322) (35.9713, 86.6328) (35.9807, 86.6334) (35.9901, 86.6342) (35.9997, 86.6349) (36.0093, 86.6357) (36.0189, 86.6366) (36.0287, 86.6376) (36.0385, 86.6386) (36.0483, 86.6397) (36.0583, 86.6408) (36.0682, 86.6421) (36.0782, 86.6433) (36.1229, 86.6488) (36.1676, 86.6539) (36.2124, 86.6584) (36.2462, 86.6618) (36.2802, 86.6648) (36.3141, 86.6676) (36.3519, 86.6707) (36.3897, 86.6734) (36.4276, 86.6758) (36.4693, 86.6785) (36.5111, 86.6808) (36.5529, 86.6827) (36.5985, 86.6848) (36.6442, 86.6864) (36.6899, 86.6877) (36.7395, 86.6891) (36.789, 86.69) (36.8386, 86.6906) (36.8921, 86.6911) (36.9456, 86.6912) (36.9991, 86.6908) (37.0564, 86.6903) (37.1138, 86.6894) (37.1711, 86.6879) (37.2324, 86.6864) (37.2936, 86.6843) (37.3548, 86.6816) (37.4198, 86.6788) (37.4849, 86.6754) (37.5499, 86.6715) (37.6188, 86.6673) (37.6877, 86.6624) (37.7565, 86.657) (37.8291, 86.6513) (37.9018, 86.6449) (37.9744, 86.6379) (38.1086, 86.6249) (38.2426, 86.6098) (38.3764, 86.5927) knots 0 0 0 0 0.057795 0.057795 0.057795 0.089038 0.089038 0.089038 0.118617 0.118617 0.118617 0.14653 0.14653 0.14653 0.172778 0.172778 0.172778 0.19736 0.19736 0.19736 0.220277 0.220277 0.220277 0.241529 0.241529 0.241529 0.261115 0.261115 0.261115 0.279036 0.279036 0.279036 0.295292 0.295292 0.295292 0.309882 0.309882 0.309882 0.329164 0.329164 0.329164 0.333477 0.333477 0.333477 0.337694 0.337694 0.337694 0.34182 0.34182 0.34182 0.345864 0.345864 0.345864 0.349834 0.349834 0.349834 0.353742 0.353742 0.353742 0.3576 0.3576 0.3576 0.361424 0.361424 0.361424 0.365232 0.365232 0.365232 0.369048 0.369048 0.369048 0.372899 0.372899 0.372899 0.376819 0.376819 0.376819 0.380853 0.380853 0.380853 0.385052 0.385052 0.385052 0.389482 0.389482 0.389482 0.394225 0.394225 0.394225 0.399381 0.399381 0.399381 0.405067 0.405067 0.405067 0.411413 0.411413 0.411413 0.418548 0.418548 0.418548 0.426565 0.426565 0.426565 0.435472 0.435472 0.435472 0.445133 0.445133 0.445133 0.45436 0.45436 0.45436 0.5 0.5 0.5 0.54564 0.54564 0.54564 0.554867 0.554867 0.554867 0.564528 0.564528 0.564528 0.573435 0.573435 0.573435 0.581452 0.581452 0.581452 0.588587 0.588587 0.588587 0.594933 0.594933 0.594933 0.600619 0.600619 0.600619 0.605775 0.605775 0.605775 0.610518 0.610518 0.610518 0.614948 0.614948 0.614948 0.619147 0.619147 0.619147 0.623181 0.623181 0.623181 0.627101 0.627101 0.627101 0.630952 0.630952 0.630952 0.634768 0.634768 0.634768 0.638576 0.638576 0.638576 0.6424 0.6424 0.6424 0.646258 0.646258 0.646258 0.650166 0.650166 0.650166 0.654136 0.654136 0.654136 0.65818 0.65818 0.65818 0.662306 0.662306 0.662306 0.666523 0.666523 0.666523 0.670836 0.670836 0.670836 0.690118 0.690118 0.690118 0.704708 0.704708 0.704708 0.720964 0.720964 0.720964 0.738885 0.738885 0.738885 0.758471 0.758471 0.758471 0.779723 0.779723 0.779723 0.80264 0.80264 0.80264 0.827222 0.827222 0.827222 0.85347 0.85347 0.85347 0.881383 0.881383 0.881383 0.910962 0.910962 0.910962 0.942205 0.942205 0.942205 1 1 1 1
  arc A259 (37.5929, 89.4495) -> (37.2281, 90.5504) centre (0.0435, 77.6158) ccw
  spline S58 degree 3 poles (36.1503, 93.3096) (36.0532, 93.216) (35.9547, 93.1238) (35.8548, 93.0333) (35.8008, 92.9843) (35.7463, 92.9358) (35.6915, 92.8878) (35.6395, 92.8423) (35.5872, 92.7973) (35.5344, 92.7528) (35.4846, 92.7108) (35.4345, 92.6692) (35.384, 92.6281) (35.3365, 92.5895) (35.2886, 92.5512) (35.2404, 92.5134) (35.1953, 92.478) (35.1499, 92.443) (35.1041, 92.4084) (35.0615, 92.3761) (35.0186, 92.3442) (34.9753, 92.3127) (34.9353, 92.2835) (34.8949, 92.2546) (34.8543, 92.2262) (34.8169, 92.1999) (34.7793, 92.174) (34.7414, 92.1484) (34.7068, 92.125) (34.6719, 92.1018) (34.6369, 92.079) (34.6051, 92.0584) (34.5731, 92.038) (34.5409, 92.0178) (34.512, 91.9998) (34.483, 91.982) (34.4538, 91.9645) (34.4152, 91.9413) (34.3763, 91.9187) (34.3372, 91.8965) (34.3285, 91.8915) (34.3197, 91.8865) (34.311, 91.8815) (34.3025, 91.8765) (34.2941, 91.8715) (34.2857, 91.8664) (34.2774, 91.8614) (34.2692, 91.8563) (34.2611, 91.8512) (34.2531, 91.8462) (34.2452, 91.841) (34.2373, 91.8359) (34.2295, 91.8308) (34.2219, 91.8256) (34.2142, 91.8204) (34.2067, 91.8152) (34.1992, 91.8099) (34.1918, 91.8046) (34.1845, 91.7994) (34.1773, 91.794) (34.1701, 91.7886) (34.163, 91.7832) (34.1559, 91.7778) (34.1489, 91.7722) (34.142, 91.7667) (34.1351, 91.761) (34.1283, 91.7553) (34.1215, 91.7496) (34.1148, 91.7437) (34.1081, 91.7378) (34.1014, 91.7318) (34.0948, 91.7257) (34.0884, 91.7195) (34.0817, 91.7132) (34.0752, 91.7067) (34.0689, 91.7002) (34.0623, 91.6934) (34.0559, 91.6865) (34.0496, 91.6795) (34.0431, 91.6722) (34.0367, 91.6647) (34.0306, 91.6571) (34.024, 91.6491) (34.0177, 91.6409) (34.0116, 91.6326) (34.0051, 91.6236) (33.9989, 91.6145) (33.9929, 91.6051) (33.9864, 91.595) (33.9803, 91.5846) (33.9745, 91.5741) (33.9682, 91.5624) (33.9623, 91.5505) (33.9569, 91.5384) (33.9509, 91.5248) (33.9455, 91.511) (33.9409, 91.497) (33.9356, 91.4812) (33.9312, 91.4651) (33.9277, 91.4488) (33.9238, 91.4305) (33.9211, 91.4119) (33.9196, 91.3932) (33.9179, 91.3725) (33.9177, 91.3517) (33.9191, 91.3309) (33.9205, 91.3084) (33.9237, 91.2859) (33.9289, 91.264) (33.9339, 91.243) (33.9406, 91.2225) (33.9478, 91.2022) (33.983, 91.1016) (34.0266, 91.0043) (34.0653, 90.9051) (34.104, 90.8059) (34.1379, 90.7049) (34.1803, 90.607) (34.1888, 90.5872) (34.1977, 90.5675) (34.2083, 90.5488) (34.2193, 90.5291) (34.2322, 90.5105) (34.2464, 90.4929) (34.2595, 90.4767) (34.2737, 90.4615) (34.289, 90.4474) (34.3028, 90.4347) (34.3174, 90.4229) (34.3327, 90.4121) (34.3462, 90.4025) (34.3604, 90.3936) (34.375, 90.3856) (34.3879, 90.3784) (34.4013, 90.3719) (34.4148, 90.366) (34.427, 90.3607) (34.4394, 90.356) (34.452, 90.3517) (34.4634, 90.3478) (34.4749, 90.3444) (34.4866, 90.3413) (34.4973, 90.3385) (34.5081, 90.336) (34.5189, 90.3339) (34.5291, 90.3318) (34.5393, 90.3301) (34.5495, 90.3286) (34.5592, 90.3272) (34.5689, 90.3261) (34.5787, 90.3251) (34.588, 90.3242) (34.5974, 90.3235) (34.6068, 90.323) (34.616, 90.3225) (34.6251, 90.3221) (34.6343, 90.3219) (34.6432, 90.3218) (34.6522, 90.3218) (34.6612, 90.3219) (34.6701, 90.322) (34.679, 90.3223) (34.6879, 90.3227) (34.6968, 90.3231) (34.7057, 90.3236) (34.7145, 90.3243) (34.7234, 90.3249) (34.7323, 90.3257) (34.7412, 90.3265) (34.7502, 90.3274) (34.7591, 90.3284) (34.768, 90.3295) (34.7771, 90.3306) (34.7861, 90.3318) (34.7952, 90.3331) (34.8043, 90.3344) (34.8135, 90.3358) (34.8226, 90.3373) (34.8319, 90.3389) (34.8412, 90.3405) (34.8505, 90.3422) (34.86, 90.3439) (34.8694, 90.3458) (34.8789, 90.3477) (34.8885, 90.3496) (34.8982, 90.3517) (34.9078, 90.3538) (34.9176, 90.356) (34.9274, 90.3582) (34.9372, 90.3605) (34.981, 90.3706) (35.025, 90.3804) (35.069, 90.3896) (35.1023, 90.3965) (35.1358, 90.403) (35.1692, 90.4093) (35.2065, 90.4163) (35.2438, 90.423) (35.2812, 90.4294) (35.3225, 90.4364) (35.3638, 90.443) (35.4051, 90.4493) (35.4503, 90.4561) (35.4955, 90.4626) (35.5409, 90.4686) (35.59, 90.4752) (35.6392, 90.4813) (35.6885, 90.487) (35.7416, 90.4931) (35.7948, 90.4988) (35.848, 90.504) (35.9051, 90.5095) (35.9623, 90.5146) (36.0194, 90.5191) (36.0805, 90.524) (36.1416, 90.5283) (36.2027, 90.5321) (36.2677, 90.5361) (36.3328, 90.5395) (36.3979, 90.5423) (36.4668, 90.5454) (36.5358, 90.5478) (36.6048, 90.5496) (36.6777, 90.5515) (36.7506, 90.5527) (36.8235, 90.5533) (36.9584, 90.5544) (37.0932, 90.5534) (37.2281, 90.5504) knots 0 0 0 0 0.057795 0.057795 0.057795 0.089038 0.089038 0.089038 0.118617 0.118617 0.118617 0.14653 0.14653 0.14653 0.172778 0.172778 0.172778 0.19736 0.19736 0.19736 0.220277 0.220277 0.220277 0.241529 0.241529 0.241529 0.261115 0.261115 0.261115 0.279036 0.279036 0.279036 0.295292 0.295292 0.295292 0.309882 0.309882 0.309882 0.329164 0.329164 0.329164 0.333477 0.333477 0.333477 0.337694 0.337694 0.337694 0.34182 0.34182 0.34182 0.345864 0.345864 0.345864 0.349834 0.349834 0.349834 0.353742 0.353742 0.353742 0.3576 0.3576 0.3576 0.361424 0.361424 0.361424 0.365232 0.365232 0.365232 0.369048 0.369048 0.369048 0.372899 0.372899 0.372899 0.376819 0.376819 0.376819 0.380853 0.380853 0.380853 0.385052 0.385052 0.385052 0.389482 0.389482 0.389482 0.394225 0.394225 0.394225 0.399381 0.399381 0.399381 0.405067 0.405067 0.405067 0.411413 0.411413 0.411413 0.418548 0.418548 0.418548 0.426565 0.426565 0.426565 0.435472 0.435472 0.435472 0.445133 0.445133 0.445133 0.45436 0.45436 0.45436 0.5 0.5 0.5 0.54564 0.54564 0.54564 0.554867 0.554867 0.554867 0.564528 0.564528 0.564528 0.573435 0.573435 0.573435 0.581452 0.581452 0.581452 0.588587 0.588587 0.588587 0.594933 0.594933 0.594933 0.600619 0.600619 0.600619 0.605775 0.605775 0.605775 0.610518 0.610518 0.610518 0.614948 0.614948 0.614948 0.619147 0.619147 0.619147 0.623181 0.623181 0.623181 0.627101 0.627101 0.627101 0.630952 0.630952 0.630952 0.634768 0.634768 0.634768 0.638576 0.638576 0.638576 0.6424 0.6424 0.6424 0.646258 0.646258 0.646258 0.650166 0.650166 0.650166 0.654136 0.654136 0.654136 0.65818 0.65818 0.65818 0.662306 0.662306 0.662306 0.666523 0.666523 0.666523 0.670836 0.670836 0.670836 0.690118 0.690118 0.690118 0.704708 0.704708 0.704708 0.720964 0.720964 0.720964 0.738885 0.738885 0.738885 0.758471 0.758471 0.758471 0.779723 0.779723 0.779723 0.80264 0.80264 0.80264 0.827222 0.827222 0.827222 0.85347 0.85347 0.85347 0.881383 0.881383 0.881383 0.910962 0.910962 0.910962 0.942205 0.942205 0.942205 1 1 1 1
  arc A260 (36.1503, 93.3096) -> (35.6723, 94.3664) centre (0.0435, 77.6158) ccw
  spline S59 degree 3 poles (34.312, 96.9978) (34.2252, 96.8946) (34.137, 96.7926) (34.0471, 96.6921) (33.9985, 96.6378) (33.9494, 96.5838) (33.8998, 96.5304) (33.8529, 96.4797) (33.8056, 96.4295) (33.7577, 96.3797) (33.7126, 96.3327) (33.6671, 96.2862) (33.6212, 96.24) (33.578, 96.1966) (33.5344, 96.1535) (33.4904, 96.1109) (33.4492, 96.0709) (33.4077, 96.0314) (33.3658, 95.9922) (33.3268, 95.9556) (33.2874, 95.9194) (33.2477, 95.8836) (33.2109, 95.8503) (33.1738, 95.8174) (33.1364, 95.7848) (33.102, 95.7548) (33.0673, 95.7251) (33.0323, 95.6957) (33.0003, 95.6688) (32.968, 95.6421) (32.9355, 95.6158) (32.9061, 95.5919) (32.8764, 95.5683) (32.8465, 95.5449) (32.8197, 95.5239) (32.7927, 95.5032) (32.7655, 95.4827) (32.7295, 95.4557) (32.6932, 95.4292) (32.6566, 95.4029) (32.6484, 95.397) (32.6403, 95.3912) (32.6321, 95.3853) (32.6242, 95.3794) (32.6163, 95.3735) (32.6085, 95.3676) (32.6008, 95.3618) (32.5932, 95.3559) (32.5856, 95.3499) (32.5782, 95.3441) (32.5709, 95.3382) (32.5636, 95.3322) (32.5564, 95.3263) (32.5493, 95.3204) (32.5422, 95.3144) (32.5353, 95.3084) (32.5284, 95.3024) (32.5216, 95.2964) (32.5149, 95.2904) (32.5083, 95.2843) (32.5017, 95.2782) (32.4952, 95.2721) (32.4887, 95.2659) (32.4824, 95.2596) (32.476, 95.2534) (32.4698, 95.2471) (32.4636, 95.2407) (32.4574, 95.2343) (32.4514, 95.2278) (32.4454, 95.2212) (32.4393, 95.2145) (32.4334, 95.2077) (32.4276, 95.2009) (32.4217, 95.1939) (32.4159, 95.1868) (32.4103, 95.1796) (32.4044, 95.1722) (32.3988, 95.1647) (32.3933, 95.1571) (32.3876, 95.1491) (32.382, 95.141) (32.3766, 95.1328) (32.371, 95.1242) (32.3656, 95.1154) (32.3604, 95.1064) (32.3548, 95.0968) (32.3496, 95.0871) (32.3446, 95.0772) (32.3392, 95.0664) (32.3342, 95.0555) (32.3296, 95.0444) (32.3245, 95.0321) (32.3199, 95.0197) (32.3158, 95.007) (32.3113, 94.9929) (32.3074, 94.9786) (32.3042, 94.9642) (32.3006, 94.9479) (32.2979, 94.9314) (32.2962, 94.9149) (32.2942, 94.8962) (32.2934, 94.8775) (32.2939, 94.8588) (32.2944, 94.838) (32.2964, 94.8172) (32.2999, 94.7967) (32.3037, 94.7745) (32.3092, 94.7525) (32.3166, 94.7312) (32.3238, 94.7109) (32.3327, 94.6912) (32.3419, 94.6717) (32.3874, 94.5753) (32.4409, 94.4831) (32.4898, 94.3885) (32.5387, 94.294) (32.583, 94.197) (32.6353, 94.1041) (32.6459, 94.0853) (32.6568, 94.0667) (32.6692, 94.0491) (32.6823, 94.0307) (32.697, 94.0135) (32.713, 93.9976) (32.7277, 93.9828) (32.7435, 93.9692) (32.7601, 93.9568) (32.7752, 93.9456) (32.7909, 93.9354) (32.8072, 93.9262) (32.8218, 93.9181) (32.8367, 93.9107) (32.8521, 93.9043) (32.8657, 93.8985) (32.8797, 93.8934) (32.8938, 93.8889) (32.9065, 93.885) (32.9193, 93.8815) (32.9322, 93.8786) (32.944, 93.8759) (32.9558, 93.8737) (32.9677, 93.8719) (32.9786, 93.8702) (32.9896, 93.8689) (33.0007, 93.8678) (33.011, 93.8669) (33.0213, 93.8662) (33.0316, 93.8658) (33.0414, 93.8655) (33.0512, 93.8653) (33.061, 93.8654) (33.0704, 93.8655) (33.0798, 93.8657) (33.0892, 93.8662) (33.0984, 93.8666) (33.1075, 93.8673) (33.1166, 93.8681) (33.1256, 93.8688) (33.1345, 93.8698) (33.1434, 93.8708) (33.1523, 93.8719) (33.1611, 93.8731) (33.1699, 93.8744) (33.1787, 93.8757) (33.1874, 93.8772) (33.1962, 93.8788) (33.205, 93.8803) (33.2137, 93.882) (33.2225, 93.8838) (33.2313, 93.8856) (33.2401, 93.8875) (33.2489, 93.8896) (33.2578, 93.8916) (33.2666, 93.8937) (33.2755, 93.896) (33.2844, 93.8982) (33.2934, 93.9006) (33.3023, 93.9031) (33.3114, 93.9056) (33.3205, 93.9081) (33.3296, 93.9108) (33.3388, 93.9135) (33.348, 93.9163) (33.3572, 93.9192) (33.3666, 93.9222) (33.376, 93.9252) (33.3853, 93.9283) (33.3948, 93.9315) (33.4043, 93.9348) (33.4139, 93.9381) (33.4564, 93.9527) (33.4991, 93.967) (33.5419, 93.9807) (33.5743, 93.9911) (33.6069, 94.0011) (33.6395, 94.0109) (33.6759, 94.0218) (33.7123, 94.0323) (33.7488, 94.0425) (33.7891, 94.0538) (33.8295, 94.0647) (33.8699, 94.0753) (33.9142, 94.0868) (33.9585, 94.0979) (34.0029, 94.1087) (34.0511, 94.1204) (34.0994, 94.1316) (34.1478, 94.1424) (34.2, 94.154) (34.2523, 94.1652) (34.3047, 94.1759) (34.3609, 94.1875) (34.4172, 94.1984) (34.4736, 94.2089) (34.5338, 94.2202) (34.5941, 94.2308) (34.6545, 94.241) (34.7188, 94.2518) (34.7831, 94.262) (34.8475, 94.2716) (34.9158, 94.2818) (34.9841, 94.2914) (35.0526, 94.3004) (35.1249, 94.3099) (35.1972, 94.3188) (35.2697, 94.327) (35.4037, 94.3422) (35.5379, 94.3553) (35.6723, 94.3664) knots 0 0 0 0 0.057795 0.057795 0.057795 0.089038 0.089038 0.089038 0.118617 0.118617 0.118617 0.14653 0.14653 0.14653 0.172778 0.172778 0.172778 0.19736 0.19736 0.19736 0.220277 0.220277 0.220277 0.241529 0.241529 0.241529 0.261115 0.261115 0.261115 0.279036 0.279036 0.279036 0.295292 0.295292 0.295292 0.309882 0.309882 0.309882 0.329164 0.329164 0.329164 0.333477 0.333477 0.333477 0.337694 0.337694 0.337694 0.34182 0.34182 0.34182 0.345864 0.345864 0.345864 0.349834 0.349834 0.349834 0.353742 0.353742 0.353742 0.3576 0.3576 0.3576 0.361424 0.361424 0.361424 0.365232 0.365232 0.365232 0.369048 0.369048 0.369048 0.372899 0.372899 0.372899 0.376819 0.376819 0.376819 0.380853 0.380853 0.380853 0.385052 0.385052 0.385052 0.389482 0.389482 0.389482 0.394225 0.394225 0.394225 0.399381 0.399381 0.399381 0.405067 0.405067 0.405067 0.411413 0.411413 0.411413 0.418548 0.418548 0.418548 0.426565 0.426565 0.426565 0.435472 0.435472 0.435472 0.445133 0.445133 0.445133 0.45436 0.45436 0.45436 0.5 0.5 0.5 0.54564 0.54564 0.54564 0.554867 0.554867 0.554867 0.564528 0.564528 0.564528 0.573435 0.573435 0.573435 0.581452 0.581452 0.581452 0.588587 0.588587 0.588587 0.594933 0.594933 0.594933 0.600619 0.600619 0.600619 0.605775 0.605775 0.605775 0.610518 0.610518 0.610518 0.614948 0.614948 0.614948 0.619147 0.619147 0.619147 0.623181 0.623181 0.623181 0.627101 0.627101 0.627101 0.630952 0.630952 0.630952 0.634768 0.634768 0.634768 0.638576 0.638576 0.638576 0.6424 0.6424 0.6424 0.646258 0.646258 0.646258 0.650166 0.650166 0.650166 0.654136 0.654136 0.654136 0.65818 0.65818 0.65818 0.662306 0.662306 0.662306 0.666523 0.666523 0.666523 0.670836 0.670836 0.670836 0.690118 0.690118 0.690118 0.704708 0.704708 0.704708 0.720964 0.720964 0.720964 0.738885 0.738885 0.738885 0.758471 0.758471 0.758471 0.779723 0.779723 0.779723 0.80264 0.80264 0.80264 0.827222 0.827222 0.827222 0.85347 0.85347 0.85347 0.881383 0.881383 0.881383 0.910962 0.910962 0.910962 0.942205 0.942205 0.942205 1 1 1 1
  circle A261 centre (0.0435, 77.6158) radius 8.89